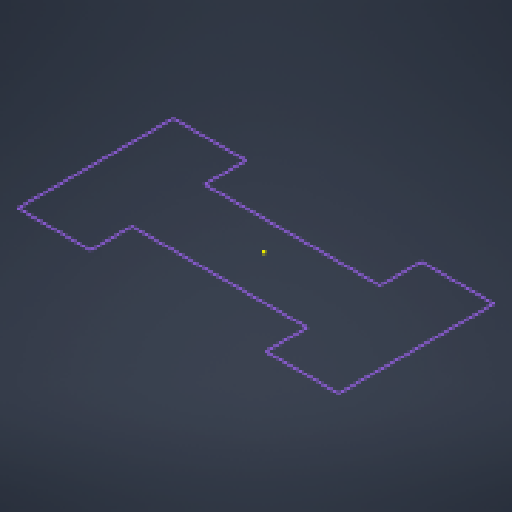
# Autodesk Inventor part: 5mm_pin
Saved by Autodesk Inventor 2026 (Build 300175050, 175E)
## iProperties
Created: 2026-04-30
Part Number: 5mm_pin
Material: Generic
Document SubType Name: Modeling
Designer: sniel
Density: 1 g/cm^3
Appearance: Default
Author: sniel
Autodesk Inventor part; units mm, degrees
ref_plane "YZ Plane" through (0, 0, 0) normal (1, 0, 0) x (0, 1, 0)
ref_plane "XZ Plane" through (0, 0, 0) normal (0, 1, 0) x (-1, 0, 0)
ref_plane "XY Plane" through (0, 0, 0) normal (0, 0, 1) x (1, 0, 0)
sketch "Sketch1" plane through (0, 0, 0) normal (0, 1, 0) x (-1, 0, 0)
  line L0 (5.3239, 5.1246) -> (5.3239, 2.6246)
  line L1 (5.3239, 2.6246) -> (-5.2761, 2.6246)
  line L2 (-5.2761, 2.6246) -> (-5.2761, 5.1246)
  line L3 (-5.2761, 5.1246) -> (-9.6761, 5.1246)
  line L4 (-9.6761, 5.1246) -> (-9.6761, -4.2754)
  line L5 (-9.6761, -4.2754) -> (-5.2761, -4.2754)
  line L6 (-5.2761, -4.2754) -> (-5.2761, -1.7754)
  line L7 (-5.2761, -1.7754) -> (5.3239, -1.7754)
  line L8 (5.3239, -1.7754) -> (5.3239, -4.2754)
  line L9 (5.3239, -4.2754) -> (9.7239, -4.2754)
  line L10 (9.7239, -4.2754) -> (9.7239, 5.1246)
  line L11 (9.7239, 5.1246) -> (5.3239, 5.1246)
  point P0 (0, 0)
  constraints: 24 end point
extrude "Extrusion1" add sketch "Sketch1" along normal blind 5
body "Solid1"
